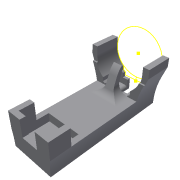
# Autodesk Inventor part: segment_1
Saved by Autodesk Inventor 2018.3 (Build 223284000, 284)
## iProperties
Created: 2020-03-08
Part Number: segment_1
Material: Generic
Document SubType Name: Modeling
Designer: Erik
Density: 1 g/cm^3
Appearance: Default
Author: Erik
Autodesk Inventor part; units mm, degrees
ref_plane "YZ Plane" through (0, 0, 0) normal (1, 0, 0) x (0, 1, 0)
ref_plane "XZ Plane" through (0, 0, 0) normal (0, 1, 0) x (-1, 0, 0)
ref_plane "XY Plane" through (0, 0, 0) normal (0, 0, 1) x (1, 0, 0)
sketch "Sketch1" plane through (0, 0, 0) normal (0, 0, 1) x (1, 0, 0)
  line L0 (-12.5, -35) -> (12.5, -35)
  line L1 (12.5, -35) -> (12.5, 35)
  line L2 (12.5, 35) -> (-12.5, 35)
  line L3 (-12.5, 35) -> (-12.5, -35)
  line L4 (-12.5, -35) -> (12.5, 35) construction
  line L5 (12.5, -35) -> (-12.5, 35) construction
  point P0 (0, 0)
  dimension "d0" = 25
  dimension "d1" = 70
  constraints: 12 end point, 2 midpoint, 2 parallel, 1 horizontal, 1 perpendicular
  measures "d0" distance of L2.end L1.end
  measures "d1" distance of L1.end L0.end
extrude "Extrusion1" add sketch "Sketch1" against normal blind 8 and the other way blind 2
sketch "Sketch2" plane through (0, 0, -8) normal (0, 0, -1) x (-1, 0, 0)
  line L0 (2.0329, -1.7) -> (-2.0329, -1.7)
  line L1 (-2.0329, 1.7) -> (2.0329, 1.7)
  line L2 (0, 0) -> (0, 0.7106)
  arc A0 (2.0329, -1.7) -> (2.0329, 1.7) centre (0, 0) ccw
  arc A1 (-2.0329, 1.7) -> (-2.0329, -1.7) centre (0, 0) ccw
  dimension "d5" = 3.4
  dimension "d6" = 90
  constraints: 6 end point, 4 point on circle, 2 centre point, 2 parallel, 1 coincident, 1 vertical
  measures "d5" distance between parallel lines of L1 L0
  measures "d6" angle of L0 L2
extrude "Extrusion2" cut sketch "Sketch2" against normal blind 9 draft -1
sketch "Sketch3" plane through (0, 0, -8) normal (0, 0, -1) x (-1, 0, 0)
  circle A0 centre (0, 0) radius 2.65
  constraints: 1 centre point, 1 coincident
extrude "Extrusion3" cut sketch "Sketch3" against normal blind 1
sketch "Sketch4" plane through (-12.5, 35, -8) normal (0, 1, 0) x (1, 0, 0)
  line L0 (16.5, 1.1622) -> (8.5, 1.1622)
  line L1 (8.5, 1.1622) -> (8.5, -17.1622)
  line L2 (8.5, -17.1622) -> (16.5, -17.1622)
  line L3 (16.5, -17.1622) -> (16.5, 1.1622)
  line L4 (16.5, 1.1622) -> (8.5, -17.1622) construction
  line L5 (8.5, 1.1622) -> (16.5, -17.1622) construction
  point P0 (12.5, -8)
  dimension "d13" = 8
  constraints: 12 end point, 2 midpoint, 2 parallel, 1 horizontal, 1 perpendicular
  measures "d13" distance of L2.end L1.end
ref_plane "Work Plane1" through (-21, 18.5, 1.5) normal (0, -1, 0) x (1, 0, 0)
extrude "Extrusion4" cut sketch "Sketch4" against normal up to surface (16.5 mm away)
sketch "Sketch5" plane through (12.5, 35, 2) normal (0, 1, 0) x (1, 0, 0)
  circle A0 centre (-12.5, -15) radius 14 projected
  line L0 (-3.95, -2.0115) -> (-3.95, -3.289) projected
  line L1 (-21.05, -3.289) -> (-21.05, -2.0115) projected
  line L2 (-19.55, 1.3) -> (-5.45, 1.3) projected
  line L3 (-19.55, 1.3) -> (-21.45, 1.3)
  circle A1 centre (-12.5, -15) radius 14.2
  line L4 (-21.45, 1.3) -> (-21.45, -3.9756)
  line L5 (-23.7628, 3.441) -> (-30.1886, -14.4304)
  line L6 (-30.1886, -14.4304) -> (-26.6886, -14.4304)
  line L7 (-23.7628, 3.441) -> (-18.2638, 3.441)
  line L8 (-18.2638, 3.441) -> (-18.2638, 1.3)
  line L9 (-12.5, 1.3) -> (-12.5, -0.8)
  line L10 (-21.25, -2.0115) -> (-21.25, -3.5376)
  line L11 (-19.75, 1.3) -> (-19.75, -1.0179)
  line L12 (-19.95, 1.3) -> (-19.95, -0.7192)
  line L13 (-19.95, -0.7192) -> (-21.45, -1.5497)
  point P0 (-12.5, 2)
  point P1 (-25, 0)
  point P2 (-28.4386, -14.4304)
  dimension "d16" = 0.2
  dimension "d18" = 90
  dimension "d23" = 3.5
  dimension "d27" = 0.2
  dimension "d28" = 0.2
  constraints: 22 end point, 5 vertical, 4 point on line, 3 horizontal, 3 point on circle, 2 midpoint, 1 centre point, 1 vertical alignment, 4 other
  measures "d16" radial gap between concentric circles of A0 A1
  measures "d18" angle of L7 L8
  measures "d23" distance of L5.end L6.end
  measures "d27" distance between parallel lines of L10 L4
  measures "d28" distance between parallel lines of L11 L12
ref_plane "Work Plane2" through (-21, 18.5, 1.5) normal (0, -1, 0) x (1, 0, 0)
extrude "Extrusion5" add sketch "Sketch5" against normal up to surface (16.5 mm away) contours L3 L4 A1 L6 L5 L7 L8 L2
sketch "Sketch6" plane through (-12.5, 35, -8) normal (0, 1, 0) x (1, 0, 0)
  line L0 (12.5, -8.7) -> (12.5, -10.8) projected
  line L1 (5.45, -8.7) -> (19.55, -8.7) projected
  line L2 (5.45, -8.7) -> (3.55, -8.7) projected
  line L3 (3.55, -8.7) -> (3.55, -13.9756) projected
  circle A0 centre (12.5, -25) radius 14.2 projected
  line L4 (5.05, -10.7192) -> (3.55, -11.5497) projected
  line L5 (5.05, -8.7) -> (5.05, -10.7192) projected
  point P0 (12.5, -8)
extrude "Extrusion6" cut sketch "Sketch6" against normal up to surface (16.5 mm away) contours L0 A0 L3 L4 L5 L2 L1 | L5 L4 L3 L2
extrude "Extrusion7" [suppressed]
mirror "Mirror1" about plane through (0, 0, 0) normal (1, 0, 0) of "Extrusion5", "Extrusion6"
fillet "Fillet1" radius 48 2 edges at (-12.5, 26.75, 2) (12.5, 26.75, 2)
extrude "Extrusion8" add sketch "Sketch6" against normal up to surface (16.5 mm away) contours L5 L4 L3 L2
mirror "Mirror2" about plane through (0, 0, 0) normal (1, 0, 0) of "Extrusion8"
sketch "Sketch7" plane through (-12.5, 35, -8) normal (0, 1, 0) x (1, 0, 0)
  line L0 (16.5, -8.7) -> (19.95, -8.7) projected
  line L1 (19.95, -8.7) -> (5.05, -8.7)
  line L2 (5.05, -8.7) -> (5.05, -7.9)
  line L3 (5.05, -7.9) -> (19.95, -7.9)
  line L4 (19.95, -7.9) -> (19.95, -8.7)
  line L5 (5.05, -10.7192) -> (5.05, -8.7) projected
  point P0 (12.5, -8)
  dimension "d33" = 0.8
  constraints: 8 end point, 2 parallel, 1 collinear, 1 horizontal, 1 perpendicular
  measures "d33" distance of L1.end L2.end
extrude "Extrusion9" cut sketch "Sketch7" against normal up to surface (16.5 mm away)
sketch "Sketch8" plane through (4, 18.5, -8) normal (-1, 0, 0) x (0, 0, 1)
  line L0 (0, 12.5923) -> (1.8919, 11.5)
  line L1 (1.8919, 11.5) -> (1.8919, 4.8744)
  line L2 (1.8919, 4.8744) -> (0, 4.0327)
  line L3 (0, 4.0327) -> (0, 12.5923)
  line L4 (0, 16.5) -> (0, -53.5) projected
  line L5 (0, 16.5) -> (7.9, 16.5) projected
  point P0 (8, -18.5)
  dimension "d48" = 5
  dimension "d49" = 120
  constraints: 8 end point, 1 collinear, 1 parallel, 1 vertical
  measures "d48" distance from line of L5 L0.end
  measures "d49" angle of L1 L0
extrude "Extrusion10" add sketch "Sketch8" along normal blind 10
sketch "Sketch9" plane through (-4, 35, -0.1) normal (1, 0, 0) x (0, 0, -1)
  line L0 (4, -2) -> (-6, -2)
  line L1 (-6, -2) -> (-6, -9)
  line L2 (-6, -9) -> (4, -9)
  line L3 (4, -9) -> (4, -2)
  line L4 (4, -2) -> (-6, -9) construction
  line L5 (-6, -2) -> (4, -9) construction
  line L6 (0, 0) -> (0, -16.5) projected
  line L7 (7.9, 0) -> (0, 0) projected
  point P0 (-0.1, -35)
  point P1 (-1, -5.5)
  dimension "d38" = 10
  dimension "d39" = 7
  dimension "d40" = 4
  dimension "d41" = 2
  constraints: 12 end point, 2 midpoint, 2 parallel, 1 horizontal, 1 perpendicular
  measures "d38" distance of L2.end L1.end
  measures "d39" distance of L1.end L0.end
  measures "d40" distance between parallel lines of L3 L6
  measures "d41" distance between parallel lines of L7 L0
extrude "Extrusion11" cut sketch "Sketch9" against normal blind 10.75
fillet "Fillet3" radius 2 2 edges at (-4, 29.5, -4.1) (0, 30, -6.1081)
fillet "Fillet4" radius 2 2 edges at (-4, 33.0461, -8) (4, 33.0461, -8)
sketch "Sketch10" plane through (0, 0, 2) normal (0, 0, 1) x (1, 0, 0)
  line L0 (-10, -16.9318) -> (10, -16.9318)
  line L1 (10, -16.9318) -> (10, -31.9318)
  line L2 (10, -31.9318) -> (-10, -31.9318)
  line L3 (-10, -31.9318) -> (-10, -16.9318)
  line L4 (-10, -16.9318) -> (10, -31.9318) construction
  line L5 (10, -16.9318) -> (-10, -31.9318) construction
  point P0 (0, 0)
  point P1 (0, -24.4318)
  dimension "d50" = 20
  dimension "d51" = 15
  constraints: 12 end point, 2 midpoint, 2 parallel, 1 horizontal, 1 perpendicular
  measures "d50" distance of L1.end L2.end
  measures "d51" distance of L0.end L1.end
extrude "Extrusion12" cut sketch "Sketch10" against normal blind 5
sketch "Sketch11" plane through (0, 0, 2) normal (0, 0, 1) x (1, 0, 0)
  line L0 (-10, -31.9318) -> (-10, -16.9318) projected
  line L1 (-10, -16.9318) -> (10, -16.9318) projected
  line L2 (10, -16.9318) -> (10, -31.9318) projected
  line L3 (10, -31.9318) -> (-10, -31.9318) projected
  line L4 (7.45, 18.5) -> (13.2349, 18.5) projected
  line L5 (7.45, 18.5) -> (-7.45, 18.5) projected
  line L6 (-7.45, 18.5) -> (-13.2349, 18.5) projected
  line L7 (-13.2349, 18.5) -> (-13.2349, -35) projected
  line L8 (-13.2349, -35) -> (13.2349, -35) projected
  line L9 (13.2349, 18.5) -> (13.2349, -35) projected
  line L10 (-10, -23.9318) -> (-13.2349, -23.9318)
  line L11 (10, -16.9318) -> (10, -31.9318) projected
  line L12 (10, -23.9318) -> (13.2349, -23.9318)
  line L13 (5, -31.9318) -> (5, -35)
  line L14 (-5, -31.9318) -> (-5, -35)
  point P0 (0, 0)
  dimension "d54" = 5
  dimension "d55" = 5
  dimension "d56" = 8
  constraints: 10 point on line, 8 end point, 2 perpendicular, 1 parallel
  measures "d54" distance between parallel lines of L14 L0
  measures "d55" distance between parallel lines of L2 L13
  measures "d56" distance between parallel lines of L3 L12
extrude "Extrusion13" add sketch "Sketch11" along normal blind 10 contours L3 L14 L8 L7 L10 L0 | L3 L2 L12 L9 L8 L13
sketch "Sketch13" plane through (14.1886, 18.5, 16.4304) normal (0, -1, 0) x (1, 0, 0)
  line L0 (-33.296, 3.4317) -> (4.9189, 3.4317)
  line L1 (4.9189, 3.4317) -> (4.9189, -3.6349)
  line L2 (4.9189, -3.6349) -> (-33.296, -3.6349)
  line L3 (-33.296, -3.6349) -> (-33.296, 3.4317)
  line L4 (-33.296, 3.4317) -> (4.9189, -3.6349) construction
  line L5 (4.9189, 3.4317) -> (-33.296, -3.6349) construction
  point P0 (-14.1886, -16.4304)
  point P1 (-14.1886, -0.1016)
  constraints: 12 end point, 2 midpoint, 2 parallel, 1 horizontal, 1 perpendicular
extrude "Extrusion14" cut sketch "Sketch13" against normal blind 1
sketch "Sketch14" plane through (14.1886, 35, 16.4304) normal (0, 0, 1) x (1, 0, 0)
  line L0 (-31.8771, -15.5) -> (-28.3771, -15.5) projected
  line L1 (-28.3771, 0) -> (-28.3771, -15.5) projected
  line L2 (-31.8771, 0) -> (-28.3771, 0) projected
  line L3 (-31.8771, 0) -> (-31.8771, -15.5) projected
  line L4 (0, -15.5) -> (3.5, -15.5) projected
  line L5 (3.5, 0) -> (3.5, -15.5) projected
  line L6 (3.5, 0) -> (0, 0) projected
  line L7 (0, 0) -> (0, -15.5) projected
  point P0 (-14.1886, -35)
extrude "Extrusion15" add sketch "Sketch14" along normal blind 5
sketch "Sketch15" plane through (0, 0, 0) normal (1, 0, 0) x (0, 1, 0)
  line L0 (18.5, 2) -> (-23.9318, 2) projected
  line L1 (15.1924, 2) -> (19.362, 14)
  line L2 (19.362, 14) -> (19.362, 17)
  line L3 (19.5, 16.4304) -> (19.5, 21.4304) projected
  line L4 (19.362, 17) -> (18.9425, 17.5751)
  line L5 (18.9425, 17.5751) -> (16.3069, 16.5205)
  line L6 (16.3069, 16.5205) -> (16.3069, 14.4082)
  line L7 (16.3069, 14.4082) -> (11.9956, 2)
  line L8 (11.9956, 2) -> (15.1924, 2)
  point P0 (0, 0)
  dimension "d64" = 3
  dimension "d65" = 12
  constraints: 14 end point, 2 parallel, 1 perpendicular, 1 point on line
  measures "d64" distance of L1.end L2.end
  measures "d65" distance from line of L0 L1.end
extrude "Extrusion16" add sketch "Sketch15" along normal mid plane 5
fillet "Fillet7" radius 5 1 edges at (0, 11.9956, 2)
fillet "Fillet8" radius 13.25 1 edges at (0, 19.362, 14)
fillet "Fillet9" radius 6.25 4 edges at (2.5, 13.594, 2) (2.5, 10.2176, 2) (-2.5, 10.2176, 2) (-2.5, 13.594, 2)
fillet "Fillet10" radius 13.5 1 edges at (0, 15.1924, 2)
fillet "Fillet11" radius 12.5 2 edges at (0, 16.3069, 16.5205) (0, 16.3069, 14.4082)
equation "\"d55\" = d54"
body "Solid1"
